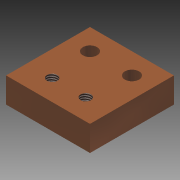
# Autodesk Inventor part: 13_0204_071
Saved by Autodesk Inventor 2012 SP1 (Build 160190100, 190)
## iProperties
Created: 2013-05-06
Part Number: 13_0204_071
Material: Default
Document SubType Name: Modeling
Designer: vogel
Density: 1 g/cm^3
Author: vogel
Autodesk Inventor part; units mm, degrees
ref_plane "YZ Plane" through (0, 0, 0) normal (1, 0, 0) x (0, 1, 0)
ref_plane "XZ Plane" through (0, 0, 0) normal (0, 1, 0) x (-1, 0, 0)
ref_plane "XY Plane" through (0, 0, 0) normal (0, 0, 1) x (1, 0, 0)
sketch "Skizze1" plane through (0, 0, 0) normal (0, 0, 1) x (1, 0, 0)
  line L0 (0, 0) -> (20, 0)
  line L1 (20, 0) -> (20, 20)
  line L2 (20, 20) -> (0, 20)
  line L3 (0, 20) -> (0, 0)
  dimension "d0" = 20
  dimension "d1" = 20
  constraints: 8 end point, 2 parallel, 1 horizontal, 1 perpendicular
  measures "d0" distance of L0.start L0.end
  measures "d1" distance of L2.end L0.start
extrude "Extrusion1" add sketch "Skizze1" along normal blind 2
sketch "Skizze2" plane through (0, 0, 2) normal (0, 0, 1) x (1, 0, 0)
  line L0 (0, 0) -> (0, 20) projected
  line L1 (20, 20) -> (20, 0) projected
  line L2 (0, 20) -> (20, 20) projected
  line L3 (0, 15) -> (20, 15)
  point P0 (5, 15)
  point P1 (15, 15)
  dimension "d4" = 5
  dimension "d5" = 5
  dimension "d6" = 10
  constraints: 4 point on line, 2 end point, 1 perpendicular
  measures "d4" distance between parallel lines of L2 L3
  measures "d5" distance from line of L0 point (5, 15)
  measures "d6" distance of point (15, 15) point (5, 15)
hole "Bohrung1" at (5, 15, 2) at (15, 15, 2) direction (0, 0, -1) diameter 3.4 end through all
sketch "Skizze3" plane through (0, 0, 2) normal (0, 0, 1) x (1, 0, 0)
  line L0 (0, 0) -> (0, 20) projected
  line L1 (20, 0) -> (0, 0) projected
  line L2 (20, 20) -> (20, 0) projected
  line L3 (0, 5) -> (20, 5)
  line L4 (10, 0) -> (10, 7.2656)
  point P0 (6, 5)
  point P1 (14, 5)
  dimension "d14" = 8
  dimension "d15" = 5
  constraints: 4 end point, 4 point on line, 2 perpendicular, 1 midpoint, 1 symmetric about line
  measures "d14" distance of point (14, 5) point (6, 5)
  measures "d15" distance between parallel lines of L3 L1
hole "Bohrung2" at (6, 5, 2) at (14, 5, 2) direction (0, 0, -1) diameter 2.459 end through all thread size "M3x0.5" class "6H" standard "ISO Metric profile"
